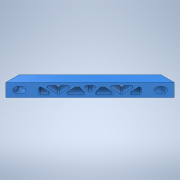
# Autodesk Inventor part: 120deg_Tslot_Gusset
Saved by Autodesk Inventor 2021 (Build 250183000, 183)
## iProperties
Created: 2020-02-22
Part Number: 120deg_Tslot_Gusset
Material: PET Plastic
Document SubType Name: Modeling
Designer: Jorian Brusind
Density: 1.541 g/cm^3
Appearance: Cyan
Author: Jorian Brusind
Autodesk Inventor part; units mm, degrees
ref_plane "YZ Plane" through (0, 0, 0) normal (1, 0, 0) x (0, 1, 0)
ref_plane "XZ Plane" through (0, 0, 0) normal (0, 1, 0) x (-1, 0, 0)
sketch "Sketch1" plane through (0, 0, 0) normal (0, 1, 0) x (-1, 0, 0)
  line L0 (9.9815, -14.535) -> (127.4857, -14.535)
  line L1 (9.9815, -14.535) -> (127.4857, -14.535) construction
  line L2 (127.4857, -14.535) -> (127.4857, 98.5548)
  line L3 (9.9815, -14.535) -> (9.9815, -4.535)
  line L4 (127.4857, 98.5548) -> (137.4841, 98.5548) construction
  line L5 (9.9815, -4.535) -> (19.9815, -4.535)
  line L6 (9.9815, -4.535) -> (-0.0185, -4.535)
  line L7 (127.4857, 92.915) -> (127.4857, 102.9692)
  line L8 (127.4857, 92.915) -> (127.4857, 122.9692)
  line L9 (127.4857, 102.9692) -> (19.9815, -4.535)
  line L10 (127.4857, 122.9692) -> (-0.0185, -4.535)
  point P0 (132.1369, 94.4644)
  dimension "d3" = 0
  dimension "d5" = 90
  dimension "d6" = 10
  dimension "d9" = 10
  dimension "d91" = 0
  dimension "d92" = 20
  dimension "d95" = 20
  constraints: 22 end point, 5 horizontal, 3 collinear, 1 parallel, 1 vertical
  measures "d3" distance between parallel lines of L0 L1
  measures "d5" angle of L2 L0
  measures "d6" distance of L0.start L3.end
  measures "d9" distance of L3.end L5.end
  measures "d91" distance between parallel lines of L7 L2
  measures "d92" distance of L8.end L7.end
  measures "d95" distance of L5.end L6.end
ref_plane "Work Plane1" through (0, 0, 15) normal (0, 0, 1) x (1, 0, 0)
extrude "Extrusion15" add sketch "Sketch1" along normal blind 20 contours L6 L10 L8 L9 L5
sketch "Sketch15" plane through (-127.4857, 0, 102.9692) normal (-1, 0, 0) x (0, 0, 1)
  circle A0 centre (10, 10) radius 2.75
  line L0 (0, 0) -> (20, 0) projected
  line L1 (20, 0) -> (20, 20) projected
  point P0 (-102.9692, 0)
  dimension "d98" = 5.5
  dimension "d99" = 10
  dimension "d100" = 10
  constraints: 1 centre point
  measures "d98" diameter of A0
  measures "d99" distance from line of L0 A0.centre
  measures "d100" distance from line of L1 A0.centre
extrude "Extrusion16" cut sketch "Sketch15" against normal through all
ref_plane "Work Plane5" through (-112.4857, 0, 102.9692) normal (-1, 0, 0) x (0, 0, 1)
sketch "Sketch17" plane through (-112.4857, 0, 102.9692) normal (-1, 0, 0) x (0, 0, 1)
  circle A0 centre (10, 10) radius 2.75 projected
  circle A1 centre (10, 10) radius 5
  point P0 (-102.9692, 0)
  dimension "d106" = 10
  constraints: 1 centre point, 1 coincident
  measures "d106" diameter of A1
extrude "Extrusion17" cut sketch "Sketch17" along normal blind 10
sketch "Sketch18" plane through (0.0185, 0, -4.535) normal (0, 0, -1) x (-1, 0, 0)
  circle A0 centre (10, 10) radius 2.75
  line L0 (0, 0) -> (20, 0) projected
  line L1 (0, 0) -> (0, 20) projected
  point P0 (0.0185, 0)
  dimension "d109" = 5.5
  dimension "d110" = 10
  dimension "d111" = 10
  constraints: 1 centre point
  measures "d109" diameter of A0
  measures "d110" distance from line of L0 A0.centre
  measures "d111" distance from line of L1 A0.centre
extrude "Extrusion18" cut sketch "Sketch18" against normal through all
ref_plane "Work Plane6" through (0.0185, 0, 10.465) normal (0, 0, -1) x (-1, 0, 0)
sketch "Sketch19" plane through (0.0185, 0, 10.465) normal (0, 0, -1) x (-1, 0, 0)
  circle A0 centre (10, 10) radius 2.75 projected
  circle A1 centre (10, 10) radius 5
  point P0 (0.0185, 0)
  dimension "d115" = 10
  constraints: 1 centre point, 1 coincident
  measures "d115" diameter of A1
extrude "Extrusion19" cut sketch "Sketch19" along normal blind 10
sketch "Sketch20" plane through (0.0185, 0, -4.535) normal (0.7071068, 0, 0.7071068) x (0.7071068, 0, -0.7071068)
  line L0 (-14.1421, 20) -> (-166.176, 20) projected
  line L1 (-90.1591, 20) -> (-90.1591, 0)
  line L2 (-14.1421, 0) -> (-166.176, 0) projected
  line L3 (-35.1591, 16) -> (-145.1591, 16)
  line L4 (-145.1591, 16) -> (-145.1591, 4)
  line L5 (-145.1591, 4) -> (-35.1591, 4)
  line L6 (-35.1591, 4) -> (-35.1591, 16)
  line L7 (-35.1591, 16) -> (-145.1591, 4) construction
  line L8 (-145.1591, 16) -> (-35.1591, 4) construction
  line L9 (-145.1591, 10) -> (-35.1591, 10)
  line L10 (-145.1591, 16) -> (-129.1591, 4)
  line L11 (-145.1591, 16) -> (-140.1591, 16)
  line L12 (-140.1591, 16) -> (-124.1591, 4)
  line L13 (-124.1591, 4) -> (-108.1591, 16)
  line L14 (-124.1591, 4) -> (-119.1591, 4)
  line L15 (-119.1591, 4) -> (-103.1591, 16)
  line L16 (-103.1591, 16) -> (-98.1591, 16)
  line L17 (-35.1591, 16) -> (-51.1591, 4)
  line L18 (-40.1591, 16) -> (-56.1591, 4)
  line L19 (-56.1591, 4) -> (-72.1591, 16)
  line L20 (-56.1591, 4) -> (-61.1591, 4)
  line L21 (-61.1591, 4) -> (-77.1591, 16)
  line L22 (-77.1591, 16) -> (-82.1591, 16)
  line L23 (-90.1591, 0) -> (-103.1591, 16)
  line L24 (-90.1591, 0) -> (-77.1591, 16)
  line L25 (-98.1591, 16) -> (-90.1591, 6.1538)
  line L26 (-90.1591, 6.1538) -> (-82.1591, 16)
  point P0 (-3.2198, 0)
  point P1 (-90.1591, 10)
  point P2 (-90.1591, 4)
  point P3 (-90.1591, 8.6154)
  point P4 (-40.1591, 16)
  point P5 (-72.1591, 16)
  point P6 (-77.1591, 16)
  point P7 (-86.9091, 4)
  point P8 (-93.4091, 4)
  dimension "d118" = 110
  dimension "d119" = 12
  dimension "d120" = 20
  dimension "d121" = 5
  dimension "d122" = 20
  dimension "d123" = 20
  dimension "d124" = 5
  dimension "d125" = 20
  dimension "d126" = 5
  constraints: 50 end point, 9 point on line, 8 midpoint, 7 symmetric about line, 3 parallel, 1 horizontal, 1 perpendicular
  measures "d118" distance of L5.end L4.end
  measures "d119" distance of L5.end L3.start
  measures "d120" distance of L3.end L10.end
  measures "d121" distance of L3.end L11.end
  measures "d122" distance of L11.end L12.end
  measures "d123" distance of L12.end L13.end
  measures "d124" distance of L12.end L14.end
  measures "d125" distance of L14.end L15.end
  measures "d126" distance of L15.end L16.end
extrude "Extrusion21" cut sketch "Sketch20" against normal through all contours L3 L26 L9 L1 | L1 L9 L25 L3 | L9 L26 L1 | L1 L25 L9 | L21 L9 L24 | L23 L9 L15 | L23 L5 L15 L9 | L9 L21 L5 L24 | L3 L18 L9 L19 | L13 L9 L12 L3 | L9 L18 L19 | L13 L12 L9 | L6 L9 L17 | L10 L9 L4 | L6 L5 L17 L9 | L9 L10 L5 L4
fillet "Fillet10" radius 2 18 edges at (-104.0889, 16, 89.5725) (-74.3904, 16, 59.874) (-56.0056, 16, 41.4892) (-48.2275, 4, 33.711) (-29.8427, 4, 15.3262) (-96.3107, 4, 81.7943) (-71.0317, 4, 56.5152) (-107.6244, 4, 93.108) (-89.2397, 4, 74.7232) (-66.4355, 4, 51.919) (-41.1564, 4, 26.64) (-29.8427, 16, 15.3262) (-107.6244, 16, 93.108) (-81.4615, 16, 66.945) (-33.3782, 16, 18.8618) (-77.9259, 16, 63.4095) (-59.5412, 16, 45.0247) (-63.0767, 16, 48.5603)
fillet "Fillet11" radius 2 1 edges at (-68.7336, 6.1538, 54.2171)
fillet "Fillet12" radius 2 2 edges at (-92.7752, 4, 78.2587) (-44.6919, 4, 30.1755)
body "Solid3"
